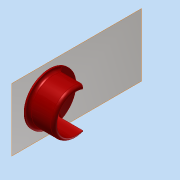
# Autodesk Inventor part: PulleyCover
Saved by Autodesk Inventor 2015 SP1 (Build 190203100, 203)
## iProperties
Created: 2015-07-03
Part Number: PulleyCover
Material: ABS Plastic
Document SubType Name: Modeling
Designer: YOUR_NAME_HERE
Density: 1.06 g/cm^3
Appearance: Smooth - Red
Author: YOUR_NAME_HERE
Autodesk Inventor part; units mm, degrees
ref_plane "YZ Plane" through (0, 0, 0) normal (1, 0, 0) x (0, 1, 0)
ref_plane "XZ Plane" through (0, 0, 0) normal (0, 1, 0) x (-1, 0, 0)
ref_plane "XY Plane" through (0, 0, 0) normal (0, 0, 1) x (1, 0, 0)
ref_plane "Work Plane2" through (0, 0, -27.25) normal (1, 0, 0) x (0, 1, 0)
sketch "Sketch5" plane through (0, 0, -27.25) normal (1, 0, 0) x (0, 1, 0)
  circle A0 centre (10.1974, 36.4793) radius 2.25 projected
  circle A1 centre (12.5, 27.25) radius 2.25 projected
  circle A2 centre (9.8332, 17.5326) radius 2.25 projected
  circle A3 centre (4.5689, 39.8851) radius 2.25 projected
  circle A4 centre (3.4977, 14.2493) radius 2.25 projected
  circle A5 centre (-4.5689, 16.6149) radius 2.25 projected
  circle A6 centre (-10.1974, 22.0207) radius 2.25 projected
  circle A7 centre (-12.5, 27.25) radius 2.25 projected
  circle A8 centre (-9.8332, 32.9674) radius 2.25 projected
  circle A9 centre (-3.4977, 38.2507) radius 2.25 projected
  circle A10 centre (0, 27.25) radius 25.4
  circle A11 centre (0, 27.25) radius 8.255
  dimension "d16" = 50.8
  dimension "d17" = 16.51
  constraints: 2 centre point, 2 coincident
  measures "d16" diameter of A10
  measures "d17" diameter of A11
extrude "Extrusion3" add sketch "Sketch5" along normal blind 1.27
sketch "Sketch6" plane through (1.27, 0, 0) normal (1, 0, 0) x (0, 0, -1)
  line L0 (-35.56, 0) -> (35.56, 0) projected
  line L1 (0, -35.56) -> (0, 35.56) projected
  circle A0 centre (0, 0) radius 19.05
  circle A1 centre (0, 0) radius 22.225
  point P0 (0, 0)
  dimension "d20" = 38.1
  dimension "d21" = 3.175
  constraints: 2 centre point, 2 coincident
  measures "d20" diameter of A0
  measures "d21" radial gap between concentric circles of A0 A1
extrude "Extrusion4" add sketch "Sketch6" along normal blind 25.4 contours A0 L1 A1 L0 | L0 A1 L1 A0 | A0 L0 A1 L1 | L1 A1 L0 A0
sketch "Sketch9" plane through (26.67, 0, 0) normal (1, 0, 0) x (0, 0, -1)
  line L0 (35.56, 0) -> (-35.56, 0) projected
  line L1 (0, 0) -> (6.5155, 17.9011) construction
  circle A0 centre (0, 0) radius 22.225 construction
  line L2 (0, 0) -> (6.5155, -17.9011) construction
  arc A1 (7.6014, -20.8847) -> (7.6014, 20.8847) centre (0, 0) ccw
  circle A2 centre (0, 0) radius 19.05 construction
  arc A3 (6.5155, -17.9011) -> (6.5155, 17.9011) centre (0, 0) ccw
  line L3 (6.5155, 17.9011) -> (7.6014, 20.8847)
  line L4 (6.5155, -17.9011) -> (7.6014, -20.8847)
  dimension "d31" = 140
  constraints: 8 end point, 6 point on circle, 2 centre point, 2 coincident, 2 collinear, 1 vertical alignment, 2 other
  measures "d31" angle of L1 L2
extrude "Extrusion7" cut sketch "Sketch9" against normal up to surface (25.4 mm away)
fillet "Fillet4" radius 3.175 1 edges at (26.67, 0, 22.225)
fillet "Fillet5" radius 3.175 3 edges at (1.27, 0, 22.225) (1.27, 19.3929, -7.0584) (1.27, -19.3929, -7.0584)
body "Solid3"
